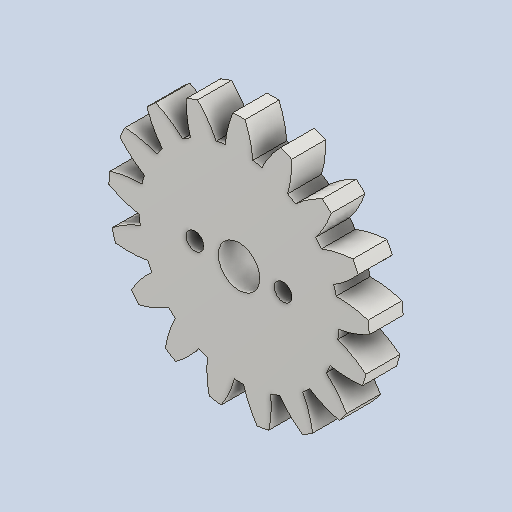
# Autodesk Inventor part: 平歯車2
Saved by Autodesk Inventor 2025.1 (Build 291241000, 241)
## iProperties
CustomPartVersion: 1
Created: 2025-05-06
Part Number: 平歯車2
Material: Steel
Document SubType Name: Modeling
Designer: yuki0520
Categories: <?xml version="1.0" encoding="UTF-16"?> <MemberInstance><Categories><FamilyTemplate><FamilyTemplateParameter ValueType="xs:double" Id="1" ObjectReferenceKey="da_z" ObjectType="kUserParameterObject"/><FamilyTemplateParameter ValueType="xs:double" Id="2" ObjectReferenceKey="da_b" ObjectType="kUserParameterObject"/><FamilyTemplateParameter ValueType="xs:double" Id="3" ObjectReferenceKey="da_beta" ObjectType="kUserParameterObject"/><FamilyTemplateParameter ValueType="xs:double" Id="4" ObjectReferenceKey="da_da" ObjectType="kUserParameterObject"/><FamilyTemplateParameter ValueType="xs:double" Id="5" ObjectReferenceKey="da_aw" ObjectType="kUserParameterObject"/><FamilyTemplateParameter ValueType="xs:string" Id="6" ObjectReferenceKey="EAIAABAAAACIAQAAAAAAAIAAAAAAAAAA" ObjectType="83910656" SubObjectId="SurfaceGeometry"/></FamilyTemplate><ParamToTemplateMap><ParamToTemplate CategoryParameter="//CategoryParameter[@InternalName='046C89C9-8512-4d59-83FE-43B91F4F132A']" TemplateParameter="1"/><ParamToTemplate CategoryParameter="//CategoryParameter[@InternalName='2552DF32-E462-4b46-AEBF-C6C7768E72AC']" TemplateParameter="2"/><ParamToTemplate CategoryParameter="//CategoryParameter[@InternalName='C9EE641D-15FC-4fae-A226-E94C4372FDD7']" TemplateParameter="3"/><ParamToTemplate><ParamToTemplate CategoryParameter="//CategoryParameter[@InternalName='00B6519A-459B-49c7-AD84-2E56D39A5744']" ConstantValue="0.100000"/></ParamToTemplate><ParamToTemplate><ParamToTemplate CategoryParameter="//CategoryParameter[@InternalName='04B31F0E-C7A6-4894-AA32-9629BEFACF47']" ConstantValue="1.000000"/></ParamToTemplate><ParamToTemplate><ParamToTemplate CategoryParameter="//CategoryParameter[@InternalName='43CBEC2E-7847-49e7-A936-2F7889FCB2D9']" ConstantValue="0.250000"/></ParamToTemplate><ParamToTemplate><ParamToTemplate CategoryParameter="//CategoryParameter[@InternalName='B1EFC894-105D-4ebd-86BF-FA20ED196853']" ConstantValue="0.350000"/></ParamToTemplate><ParamToTemplate><ParamToTemplate CategoryParameter="//CategoryParameter[@InternalName='51175063-3D10-4879-93E8-6246FE8B403D']" ConstantValue="2060000000.000000"/></ParamToTemplate><ParamToTemplate><ParamToTemplate CategoryParameter="//CategoryParameter[@InternalName='A3A52E27-4454-46a9-B0BD-C932399B70AF']" ConstantValue="0.300000"/></ParamToTemplate><ParamToTemplate><ParamToTemplate CategoryParameter="//CategoryParameter[@InternalName='91B76062-C214-41d9-B1B9-14D2AB99603D']" ConstantValue="0.200000"/></ParamToTemplate><ParamToTemplate><ParamToTemplate CategoryParameter="//CategoryParameter[@InternalName='374E806E-8B8A-4dda-A9AA-1039D6500AD2']" ConstantValue="5.000000"/></ParamToTemplate><ParamToTemplate><ParamToTemplate CategoryParameter="//CategoryParameter[@InternalName='2D373A89-B862-43d6-8D0B-0CBF12AB9F6C']" ConstantValue="0.349066"/></ParamToTemplate><ParamToTemplate CategoryParameter="//CategoryParameter[@InternalName='37777632-D6A2-4fac-9D53-DB8ACD95C989']" TemplateParameter="4"/><ParamToTemplate CategoryParameter="//CategoryParameter[@InternalName='FD1017F1-B727-4f7e-9707-0F86F1FF9423']" TemplateParameter="5"/><ParamToTemplate><ParamToTemplate CategoryParameter="//CategoryParameter[@InternalName='9E1B4470-B2D3-4ff1-B813-535BB4CDF51A']" ConstantValue="3520000.000000"/></ParamToTemplate><ParamToTemplate><ParamToTemplate CategoryParameter="//CategoryParameter[@InternalName='F8452263-BFF6-458c-9FB1-07C4B99E95CD']" ConstantValue="11400000.000000"/></ParamToTemplate><ParamToTemplate><ParamToTemplate CategoryParameter="//CategoryParameter[@InternalName='3E3BB259-FD49-497f-8171-6EBC954A3479']" ConstantValue="2.000000"/></ParamToTemplate><ParamToTemplate CategoryParameter="//CategoryParameter[@InternalName='27C3BAF2-7550-4e4b-AE2C-0DB134B7D9B7']" TemplateParameter="6"/></ParamToTemplateMap><Category DisplayName="Gear" InternalName="DC85795E-93AB-48d5-8EEE-5A27447B64BD" Mnemonic="Gear"><CategoryParameter DisplayName="z" InternalName="046C89C9-8512-4d59-83FE-43B91F4F132A" Mnemonic="z"/><CategoryParameter DisplayName="b" InternalName="2552DF32-E462-4b46-AEBF-C6C7768E72AC" Mnemonic="b"/><CategoryParameter DisplayName="||b|" InternalName="C9EE641D-15FC-4fae-A226-E94C4372FDD7" Mnemonic="beta"/><CategoryParameter DisplayName="x" InternalName="00B6519A-459B-49c7-AD84-2E56D39A5744" Mnemonic="x"/><CategoryParameter DisplayName="a*" InternalName="04B31F0E-C7A6-4894-AA32-9629BEFACF47" Mnemonic="a"/><CategoryParameter DisplayName="c*" InternalName="43CBEC2E-7847-49e7-A936-2F7889FCB2D9" Mnemonic="c"/><CategoryParameter DisplayName="r|.f|*" InternalName="B1EFC894-105D-4ebd-86BF-FA20ED196853" Mnemonic="rf"/><CategoryParameter DisplayName="E" InternalName="51175063-3D10-4879-93E8-6246FE8B403D" Mnemonic="E"/><CategoryParameter DisplayName="||m|" InternalName="A3A52E27-4454-46a9-B0BD-C932399B70AF" Mnemonic="mi"/><Category DisplayName="SpurGear" InternalName="26C5A22E-A91E-4dfd-A3B3-23CCAFAE1764" Mnemonic="SpurGear"><CategoryParameter DisplayName="m" InternalName="91B76062-C214-41d9-B1B9-14D2AB99603D" Mnemonic="m"/><CategoryParameter DisplayName="P" InternalName="374E806E-8B8A-4dda-A9AA-1039D6500AD2" Mnemonic="PP"/><CategoryParameter DisplayName="||a|" InternalName="2D373A89-B862-43d6-8D0B-0CBF12AB9F6C" Mnemonic="alpha"/><CategoryParameter DisplayName="d|.a|" InternalName="37777632-D6A2-4fac-9D53-DB8ACD95C989" Mnemonic="da"/><CategoryParameter DisplayName="a|.w|" InternalName="FD1017F1-B727-4f7e-9707-0F86F1FF9423" Mnemonic="aw"/><CategoryParameter DisplayName="||s||.Flim|" InternalName="9E1B4470-B2D3-4ff1-B813-535BB4CDF51A" Mnemonic="sFlim"/><CategoryParameter DisplayName="||s||.Hlim|" InternalName="F8452263-BFF6-458c-9FB1-07C4B99E95CD" Mnemonic="sHlim"/><CategoryParameter DisplayName="タイプ" InternalName="3E3BB259-FD49-497f-8171-6EBC954A3479" Mnemonic="type"/><CategoryParameter DisplayName="PitchDiameter" InternalName="27C3BAF2-7550-4e4b-AE2C-0DB134B7D9B7" Mnemonic="IDS_PITCHDIAM"/></Category></Category></Categories></MemberInstance>
Density: 1 g/cm^3
Appearance: Steel
Author: yuki0520
Autodesk Inventor part; units mm, degrees
sketch "Sketch1" plane through (0, 0, 0) normal (0, 0, 1) x (1, 0, 0)
  circle A0 centre (0, 0) radius 19.2
  dimension "d0" = 38.4
  constraints: 1 centre point
  measures "d0" diameter of A0
extrude "Extrusion1" add sketch "Sketch1" along normal blind 5
ref_plane "Work Plane2" through (0, 0, 2.5) normal (0, 0, 1) x (1, 0, 0)
sketch "Sketch2" plane through (0, 0, 0) normal (0, 0, -1) x (-1, 0, 0)
  circle A0 centre (0, 0) radius 19.2 projected
  circle A1 centre (0, 0) radius 17
  dimension "d3" = 34
  constraints: 1 centre point, 1 coincident
  measures "d3" diameter of A1
surface extrude "ピッチ円直径" sketch "Sketch2" against normal through all shown no curves A1
ref_plane "Work Plane8" through (0, 0, 0) normal (0.9829731, 0.1837495, 0) x (0, 0, 1)
ref_plane "Work Plane9" through (0, 0, 0) normal (1, 0, 0) x (0, 1, 0)
spur gear teeth "平歯車" teeth 17 pitch diameter 34 tip diameter 38.4 root diameter 29.4 face width 5 start plane through (0, 0, 0) normal (0, 0, -1) x (-1, 0, 0)
sketch "スケッチ3" plane through (0, 0, 5) normal (0, 0, 1) x (1, 0, 0)
  arc A0 (-6.1016, 18.2047) -> (-7.7553, 17.564) centre (0, 0) ccw projected
  arc A1 (-7.7553, 17.564) -> (-7.1531, 12.8422) centre (7.4056, 17.0983) ccw projected
  arc A2 (-7.1531, 12.8422) -> (-8.3075, 12.1275) centre (0, 0) ccw projected
  arc A3 (-8.3075, 12.1275) -> (-12.2659, 14.7712) centre (-18.6067, 0.9921) ccw projected
  arc A4 (-12.2659, 14.7712) -> (-13.5765, 13.5765) centre (0, 0) ccw projected
  arc A5 (-13.5765, 13.5765) -> (-11.3092, 9.391) centre (0.7289, 18.6189) ccw projected
  arc A6 (-11.3092, 9.391) -> (-12.1275, 8.3075) centre (0, 0) ccw projected
  arc A7 (-12.1275, 8.3075) -> (-16.7735, 9.3428) centre (-17.7087, -5.7964) ccw projected
  arc A8 (-16.7735, 9.3428) -> (-17.564, 7.7553) centre (0, 0) ccw projected
  arc A9 (-17.564, 7.7553) -> (-13.938, 4.6715) centre (-6.0462, 17.6249) ccw projected
  arc A10 (-13.938, 4.6715) -> (-14.3095, 3.3656) centre (0, 0) ccw projected
  arc A11 (-14.3095, 3.3656) -> (-19.0159, 2.6526) centre (-14.4189, -11.8021) ccw projected
  arc A12 (-19.0159, 2.6526) -> (-19.1795, 0.8867) centre (0, 0) ccw projected
  arc A13 (-19.1795, 0.8867) -> (-14.6843, -0.6789) centre (-12.0048, 14.2506) ccw projected
  arc A14 (-14.6843, -0.6789) -> (-14.559, -2.0309) centre (0, 0) ccw projected
  arc A15 (-14.559, -2.0309) -> (-18.69, -4.3959) centre (-9.1819, -16.2138) ccw projected
  arc A16 (-18.69, -4.3959) -> (-18.2047, -6.1016) centre (0, 0) ccw projected
  arc A17 (-18.2047, -6.1016) -> (-13.4475, -5.9376) centre (-16.3421, 8.9517) ccw projected
  arc A18 (-13.4475, -5.9376) -> (-12.8422, -7.1531) centre (0, 0) ccw projected
  arc A19 (-12.8422, -7.1531) -> (-15.84, -10.8506) centre (-2.7047, -18.4358) ccw projected
  arc A20 (-15.84, -10.8506) -> (-14.7712, -12.2659) centre (0, 0) ccw projected
  arc A21 (-14.7712, -12.2659) -> (-10.3945, -10.3945) centre (-18.4722, 2.4437) ccw projected
  arc A22 (-10.3945, -10.3945) -> (-9.391, -11.3092) centre (0, 0) ccw projected
  arc A23 (-9.391, -11.3092) -> (-10.8506, -15.84) centre (4.1377, -18.168) ccw projected
  arc A24 (-10.8506, -15.84) -> (-9.3428, -16.7735) centre (0, 0) ccw projected
  arc A25 (-9.3428, -16.7735) -> (-5.9376, -13.4475) centre (-18.1076, -4.3942) ccw projected
  arc A26 (-5.9376, -13.4475) -> (-4.6715, -13.938) centre (0, 0) ccw projected
  arc A27 (-4.6715, -13.938) -> (-4.3959, -18.69) centre (10.4213, -15.4464) ccw projected
  arc A28 (-4.3959, -18.69) -> (-2.6526, -19.0159) centre (0, 0) ccw projected
  arc A29 (-2.6526, -19.0159) -> (-0.6789, -14.6843) centre (-15.2975, -10.6387) ccw projected
  arc A30 (-0.6789, -14.6843) -> (0.6789, -14.6843) centre (0, 0) ccw projected
  arc A31 (0.6789, -14.6843) -> (2.6526, -19.0159) centre (15.2975, -10.6387) ccw projected
  arc A32 (2.6526, -19.0159) -> (4.3959, -18.69) centre (0, 0) ccw projected
  arc A33 (4.3959, -18.69) -> (4.6715, -13.938) centre (-10.4213, -15.4464) ccw projected
  arc A34 (4.6715, -13.938) -> (5.9376, -13.4475) centre (0, 0) ccw projected
  arc A35 (5.9376, -13.4475) -> (9.3428, -16.7735) centre (18.1076, -4.3942) ccw projected
  arc A36 (9.3428, -16.7735) -> (10.8506, -15.84) centre (0, 0) ccw projected
  arc A37 (10.8506, -15.84) -> (9.391, -11.3092) centre (-4.1377, -18.168) ccw projected
  arc A38 (9.391, -11.3092) -> (10.3945, -10.3945) centre (0, 0) ccw projected
  arc A39 (10.3945, -10.3945) -> (14.7712, -12.2659) centre (18.4722, 2.4437) ccw projected
  arc A40 (14.7712, -12.2659) -> (15.84, -10.8506) centre (0, 0) ccw projected
  arc A41 (15.84, -10.8506) -> (12.8422, -7.1531) centre (2.7047, -18.4358) ccw projected
  arc A42 (12.8422, -7.1531) -> (13.4475, -5.9376) centre (0, 0) ccw projected
  arc A43 (13.4475, -5.9376) -> (18.2047, -6.1016) centre (16.3421, 8.9517) ccw projected
  arc A44 (18.2047, -6.1016) -> (18.69, -4.3959) centre (0, 0) ccw projected
  arc A45 (18.69, -4.3959) -> (14.559, -2.0309) centre (9.1819, -16.2138) ccw projected
  arc A46 (14.559, -2.0309) -> (14.6843, -0.6789) centre (0, 0) ccw projected
  arc A47 (14.6843, -0.6789) -> (19.1795, 0.8867) centre (12.0048, 14.2506) ccw projected
  arc A48 (19.1795, 0.8867) -> (19.0159, 2.6526) centre (0, 0) ccw projected
  arc A49 (19.0159, 2.6526) -> (14.3095, 3.3656) centre (14.4189, -11.8021) ccw projected
  arc A50 (14.3095, 3.3656) -> (13.938, 4.6715) centre (0, 0) ccw projected
  arc A51 (13.938, 4.6715) -> (17.564, 7.7553) centre (6.0462, 17.6249) ccw projected
  arc A52 (17.564, 7.7553) -> (16.7735, 9.3428) centre (0, 0) ccw projected
  arc A53 (16.7735, 9.3428) -> (12.1275, 8.3075) centre (17.7087, -5.7964) ccw projected
  arc A54 (12.1275, 8.3075) -> (11.3092, 9.391) centre (0, 0) ccw projected
  arc A55 (11.3092, 9.391) -> (13.5765, 13.5765) centre (-0.7289, 18.6189) ccw projected
  arc A56 (13.5765, 13.5765) -> (12.2659, 14.7712) centre (0, 0) ccw projected
  arc A57 (12.2659, 14.7712) -> (8.3075, 12.1275) centre (18.6067, 0.9921) ccw projected
  arc A58 (8.3075, 12.1275) -> (7.1531, 12.8422) centre (0, 0) ccw projected
  arc A59 (7.1531, 12.8422) -> (7.7553, 17.564) centre (-7.4056, 17.0983) ccw projected
  arc A60 (7.7553, 17.564) -> (6.1016, 18.2047) centre (0, 0) ccw projected
  arc A61 (6.1016, 18.2047) -> (3.3656, 14.3095) centre (16.9919, 7.6467) ccw projected
  arc A62 (3.3656, 14.3095) -> (2.0309, 14.559) centre (0, 0) ccw projected
  arc A63 (2.0309, 14.559) -> (0.8867, 19.1795) centre (-13.0822, 13.2685) ccw projected
  arc A64 (0.8867, 19.1795) -> (-0.8867, 19.1795) centre (0, 0) ccw projected
  arc A65 (-0.8867, 19.1795) -> (-2.0309, 14.559) centre (13.0822, 13.2685) ccw projected
  arc A66 (-2.0309, 14.559) -> (-3.3656, 14.3095) centre (0, 0) ccw projected
  arc A67 (-3.3656, 14.3095) -> (-6.1016, 18.2047) centre (-16.9919, 7.6467) ccw projected
  circle A68 centre (0, 0) radius 3.05
  circle A69 centre (0, 0) radius 6.5
  circle A70 centre (6.5, 0) radius 1.3
  line L0 (-6.5, 0) -> (6.5, 0)
  circle A71 centre (-6.5, 0) radius 1.3
  dimension "d49" = 6.1
  dimension "d50" = 13
  dimension "d51" = 2.6
  dimension "d52" = 2.6
  constraints: 4 centre point, 2 coincident, 2 end point, 2 point on circle, 1 horizontal, 1 midpoint
  measures "d49" diameter of A68
  measures "d50" diameter of A69
  measures "d51" diameter of A70
  measures "d52" diameter of A71
extrude "押し出し2" cut sketch "スケッチ3" against normal blind 10 contours L0 A68 | A68 L0 | L0 A69 A70 | A70 A69 L0 | A71 A69 L0 | L0 A69 A71 | A70 A69 | A69 A71
equation "\"d0\" = da_da"
equation "\"d1\" = da_b"
equation "\"d52\" = d51"
equation "\"d3\" = da_d"
equation "\"d16\" = da_aw"
equation "\"d43\" = da_aw"
equation "\"d46\" = da_aw"
equation "\"da_da\" = 38.4"
equation "\"da_b\" = 5"
equation "\"da_d\" = 34"
equation "\"da_aw\" = 34"
body "Solid1"
body "Srf1"
